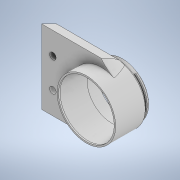
# Autodesk Inventor part: Adapter_Remington_v2
Saved by Autodesk Inventor 2020 (Build 240168000, 168)
## iProperties
Created: 2019-09-16
Part Number: Adapter_Remington_v2
Material: Generic
Document SubType Name: Modeling
Designer: rainer
Density: 1 g/cm^3
Appearance: Default
Author: rainer
Autodesk Inventor part; units mm, degrees
ref_plane "XZ Plane" through (0, 0, 0) normal (0, 1, 0) x (-1, 0, 0)
ref_plane "XY Plane" through (0, 0, 0) normal (0, 0, 1) x (1, 0, 0)
sketch "Sketch1" plane through (0, 0, 0) normal (0, 0, 1) x (1, 0, 0)
  circle A0 centre (0, 0) radius 19.75
  dimension "d0" = 39.5
  constraints: 1 centre point, 1 coincident
  measures "d0" diameter of A0
extrude "Extrusion1" add sketch "Sketch1" along normal blind 20
sketch "Sketch2" plane through (0, 0, 0) normal (0, 0, -1) x (-1, 0, 0)
  circle A0 centre (0, 0) radius 17.5
  dimension "d3" = 35
  constraints: 1 centre point, 1 coincident
  measures "d3" diameter of A0
extrude "Extrusion2" add sketch "Sketch2" along normal blind 4.4
sketch "Sketch3" plane through (0, 0, 0) normal (0, 0, -1) x (-1, 0, 0)
  circle A0 centre (0, 0) radius 18.35
  dimension "d6" = 36.7
  constraints: 1 centre point, 1 coincident
  measures "d6" diameter of A0
extrude "Extrusion3" add sketch "Sketch3" along normal blind 1.5
sketch "Sketch4" plane through (0, 0, -4.4) normal (0, 0, -1) x (-1, 0, 0)
  circle A0 centre (0, 0) radius 18.2
  dimension "d9" = 36.4
  constraints: 1 centre point, 1 coincident
  measures "d9" diameter of A0
extrude "Extrusion4" add sketch "Sketch4" against normal blind 2
ref_plane "Work Plane2" through (0, 0, -4.4) normal (0, 0, -1) x (-1, 0, 0)
sketch "Sketch5" plane through (0, 0, -4.4) normal (0, 0, -1) x (-1, 0, 0)
  circle A0 centre (0, 0) radius 16.5
  dimension "d13" = 33
  constraints: 1 centre point, 1 coincident
  measures "d13" diameter of A0
extrude "Extrusion5" cut sketch "Sketch5" against normal through all
ref_plane "Work Plane1" through (-40, 0, 0) normal (1, 0, 0) x (0, 1, 0)
sketch "Sketch6" plane through (-40, 0, 0) normal (1, 0, 0) x (0, 1, 0)
  line L0 (-20, 0) -> (20, 0)
  line L1 (20, 0) -> (20, 10)
  line L2 (20, 10) -> (-20, 10)
  line L3 (-20, 10) -> (-20, 0)
  line L4 (19.75, 0) -> (-19.75, 0) projected
  point P0 (0, 0)
  point P1 (0, 10)
  dimension "d17" = 10
  dimension "d18" = 40
  dimension "d21" = 0
  constraints: 8 end point, 2 parallel, 1 horizontal, 1 midpoint, 1 perpendicular, 1 vertical alignment
  measures "d17" distance of L0.end L1.end
  measures "d18" distance of L1.end L2.end
  measures "d21" distance between parallel lines of L4 L0
extrude "Extrusion6" add sketch "Sketch6" along normal blind 23
sketch "Sketch7" plane through (0, 0, 0) normal (0, 0, -1) x (-1, 0, 0)
  line L0 (40, -20) -> (40, 20) projected
  line L1 (40, -20) -> (17, -20) projected
  line L2 (40, 20) -> (17, 20) projected
  point P0 (0, 0)
  point P1 (32.5, -10)
  point P2 (32.5, 10)
  dimension "d22" = 7.5
  dimension "d23" = 10
  dimension "d24" = 10
  measures "d22" distance from line of L0 point (32.5, -10)
  measures "d23" distance from line of L1 point (32.5, -10)
  measures "d24" distance from line of L2 point (32.5, 10)
hole "Hole1" at (-32.5, -10, 0) at (-32.5, 10, 0) direction (0, 0, 1) diameter 4.4 end through all counterbore diameter 8 counterbore depth 5
thicken "Thicken1" operation add thickness 2.8 both sides no extend neighbours yes toward (0, 0, 1) faces at (18.3155, -2.8917, 20)
thicken "Thicken2" operation add thickness 0.1 both sides no extend neighbours yes toward (0, 0, 1) faces at (18.3155, -2.8917, 22.8)
sketch "Sketch8" plane through (0, 0, 22.9) normal (0, 0, 1) x (1, 0, 0)
  circle A0 centre (0, 0) radius 18.75
  dimension "d36" = 37.5
  constraints: 1 centre point, 1 coincident
  measures "d36" diameter of A0
extrude "Extrusion7" cut sketch "Sketch8" against normal blind 20
thicken "Thicken3" operation add thickness 3 both sides no extend neighbours yes toward (0, 0, -1) faces at (19.2254, -1.5755, 22.9)
sketch "Sketch9" plane through (-40, 0, 0) normal (-1, 0, 0) x (0, 0, 1)
  line L0 (10, -20) -> (0, -20) projected
  line L1 (10, -20) -> (10, -25)
  line L2 (10, -20) -> (15, -20) construction
  line L3 (10, -25) -> (0, -20)
  line L4 (0, -20) -> (10, -20)
  line L5 (0, 20) -> (10, 20) projected
  line L6 (10, 20) -> (10, 25)
  line L7 (10, 20) -> (15, 20) construction
  line L8 (10, 25) -> (0, 20)
  line L9 (0, 20) -> (10, 20)
  point P0 (0, 0)
  dimension "d42" = 5
  dimension "d43" = 90
  dimension "d44" = 5
  dimension "d45" = 90
  constraints: 16 end point, 3 perpendicular, 2 horizontal, 2 vertical, 1 collinear
  measures "d42" distance of L0.start L1.end
  measures "d43" angle of L1 L2
  measures "d44" distance of L5.end L6.end
  measures "d45" angle of L7 L6
extrude "Extrusion8" add sketch "Sketch9" against normal blind 23
thicken "Thicken4" operation add thickness 17 both sides no extend neighbours yes toward (1, 0, 0) faces at (-17, 18.351, 6.6667)
thicken "Thicken5" operation add thickness 17 both sides no extend neighbours yes toward (1, 0, 0) faces at (-17, -18.351, 6.6667)
fillet "Fillet3" radius 20 1 edges at (0, 19.75, 5)
fillet "Fillet4" radius 20 1 edges at (0, -19.75, 5)
sketch "Sketch10" plane through (0, 0, -4.4) normal (0, 0, -1) x (-1, 0, 0)
  circle A0 centre (0, 0) radius 17.5
  circle A1 centre (0, 0) radius 18.2 projected
  circle A2 centre (0, 0) radius 18
  line L0 (-10, -31.5176) -> (10, -31.5176)
  line L1 (10, -31.5176) -> (10, 31.5176)
  line L2 (10, 31.5176) -> (-10, 31.5176)
  line L3 (-10, 31.5176) -> (-10, -31.5176)
  point P0 (-10, 0)
  point P1 (0, -31.5176)
  point P2 (-10, 15.2066)
  point P3 (-10, 14.3614)
  point P4 (10, 14.3614)
  point P5 (10, 15.2066)
  point P6 (-10, -14.3614)
  point P7 (-10, -15.2066)
  point P8 (10, -15.2066)
  point P9 (10, -14.3614)
  dimension "d54" = 35
  dimension "d55" = 36
  dimension "d56" = 20
  constraints: 8 end point, 2 centre point, 2 coincident, 2 midpoint, 2 parallel, 1 horizontal, 1 horizontal alignment, 1 perpendicular, 1 vertical alignment
  measures "d54" diameter of A0
  measures "d55" diameter of A2
  measures "d56" distance of L0.start L0.end
extrude "Extrusion9" cut sketch "Sketch10" against normal up to surface (2.9 mm away) contours A0 L3 A2 L1 | L1 A2 L3 A0 | A2 L3 A1 L1 | L1 A1 L3 A2
fillet "Fillet5" radius 0.5 10 edges at (18.2, 0, -4.4) (18.2, 0, -2.4) (-16.0194, -8.6383, -2.4) (-16.0194, 8.6383, -2.4) (-16.0194, -8.6383, -4.4) (-16.0194, 8.6383, -4.4) (10, -15.2066, -3.4) (10, 15.2066, -3.4) (-10, 15.2066, -3.4) (-10, -15.2066, -3.4)
chamfer "Chamfer1" distance 2.25 angle 82 1 edges at (-18.75, 0, 2.9) measured on face at (-18.25, 0, 2.9)
body "Solid1"
